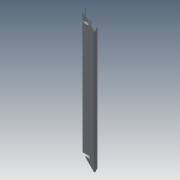
# Autodesk Inventor part: leg
Saved by Autodesk Inventor 2015 (Build 190159000, 159)
## iProperties
Created: 2014-09-01
Part Number: leg
Material: Generic
Document SubType Name: Modeling
Designer: shohei
Density: 1 g/cm^3
Appearance: Default
Author: shohei
Autodesk Inventor part; units mm, degrees
ref_plane "YZ Plane" through (0, 0, 0) normal (1, 0, 0) x (0, 1, 0)
ref_plane "XZ Plane" through (0, 0, 0) normal (0, 1, 0) x (-1, 0, 0)
ref_plane "XY Plane" through (0, 0, 0) normal (0, 0, 1) x (1, 0, 0)
sketch "Sketch2" plane through (0, 0, 0) normal (0, 1, 0) x (-1, 0, 0)
  line L0 (0, 0) -> (40, 0)
  line L1 (40, 0) -> (40, 460)
  line L2 (40, 460) -> (0, 460)
  line L3 (0, 460) -> (0, 0)
  line L4 (40, 430) -> (20, 430)
  line L5 (20, 430) -> (20, 421)
  line L6 (20, 421) -> (40, 421)
  line L7 (40, 421) -> (40, 430)
  line L8 (40, 39) -> (15, 39)
  line L9 (15, 39) -> (15, 30)
  line L10 (15, 30) -> (40, 30)
  line L11 (40, 30) -> (40, 39)
  dimension "d25" = 40
  dimension "d31" = 9
  dimension "d32" = 20
  dimension "d33" = 30
  dimension "d38" = 30
  dimension "d39" = 9
  dimension "d40" = 25
  dimension "d43" = 400
  constraints: 24 end point, 6 parallel, 3 horizontal, 3 perpendicular, 2 point on line
  measures "d25" distance of L1.end L2.end
  measures "d31" distance of L4.end L5.end
  measures "d32" distance of L5.end L6.end
  measures "d33" distance between parallel lines of L2 L4
  measures "d38" distance between parallel lines of L0 L10
  measures "d39" distance of L8.end L9.end
  measures "d40" distance between parallel lines of L1 L9
  measures "d43" distance between parallel lines of L4 L10
extrude "Extrusion5" add sketch "Sketch2" along normal blind 9 contours L3 L2 L1 L4 L5 L6 L8 L9 L10 L0
body "Solid5"
